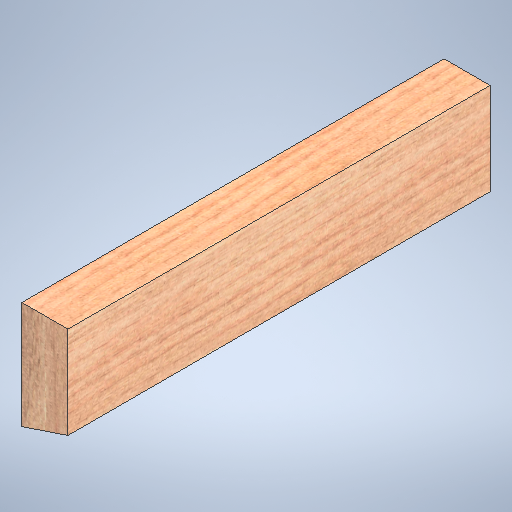
# Autodesk Inventor part: Ceiling_Support
Saved by Autodesk Inventor 2025 (Build 290162010, 162A)
## iProperties
Created: 2024-09-15
Part Number: Ceiling_Support
Material: Wood (Birch)
Document SubType Name: Modeling
Designer: Tom
Density: 0.55 g/cm^3
Appearance: Birch - Natural Polished
Author: Tom
Autodesk Inventor part; units mm, degrees
ref_plane "YZ Plane" through (0, 0, 0) normal (1, 0, 0) x (0, 1, 0)
ref_plane "XZ Plane" through (0, 0, 0) normal (0, 1, 0) x (-1, 0, 0)
ref_plane "XY Plane" through (0, 0, 0) normal (0, 0, 1) x (1, 0, 0)
sketch "Sketch1" plane through (0, 0, 0) normal (0, 0, 1) x (1, 0, 0)
  line L0 (0, 0) -> (3263.9, 1089.025)
  line L1 (0, 0) -> (-88.9, 0)
  line L2 (38.1, 12.7124) -> (38.1, 88.9)
  line L3 (38.1, 88.9) -> (0, 88.9)
  line L4 (0, 88.9) -> (0, 0)
  dimension "d33" = 1089.025
  dimension "d36" = 3352.8
  dimension "d37" = 88.9
  dimension "d38" = 88.9
  dimension "d39" = 38.1
  constraints: 10 end point, 2 coincident, 2 vertical, 1 horizontal, 1 perpendicular, 1 point on line
  measures "d33" vertical distance of L0.end point (0, 0)
  measures "d36" horizontal distance of L1.end L0.end
  measures "d37" distance of point (0, 0) L1.end
  measures "d38" distance of L3.end L4.end
  measures "d39" distance of L2.end L3.end
extrude "Extrusion2" add sketch "Sketch1" along normal blind 349.25
body "Solid2"
